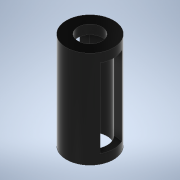
# Autodesk Inventor part: attachmentcustom
Saved by Autodesk Inventor 2022 (Build 260153000, 153)
## iProperties
Created: 2020-10-27
Part Number: attachmentcustom
Material: PET Plastic
Document SubType Name: Modeling
Designer: juanp
Density: 1.541 g/cm^3
Appearance: Polycarbonate - Clear
Author: juanp
Autodesk Inventor part; units mm, degrees
ref_plane "YZ Plane" through (0, 0, 0) normal (1, 0, 0) x (0, 1, 0)
ref_plane "XZ Plane" through (0, 0, 0) normal (0, 1, 0) x (-1, 0, 0)
ref_plane "XY Plane" through (0, 0, 0) normal (0, 0, 1) x (1, 0, 0)
sketch "Sketch6" plane through (0, 0, 0) normal (0, 1, 0) x (-1, 0, 0)
  circle A0 centre (0, 0) radius 8.75
  circle A1 centre (0, 0) radius 4.5
  dimension "d18" = 17.5
  dimension "d35" = 9
  constraints: 2 centre point, 2 coincident
  measures "d18" diameter of A0
  measures "d35" diameter of A1
extrude "Extrusion5" add sketch "Sketch6" along normal blind 36
sketch "Sketch10" plane through (0, 0, 0) normal (0, -1, 0) x (1, 0, 0)
  circle A0 centre (0, 0) radius 6.35
  dimension "d32" = 12.7
  constraints: 1 centre point, 1 coincident
  measures "d32" diameter of A0
extrude "Extrusion8" cut sketch "Sketch10" against normal blind 32.6
sketch "Sketch11" plane through (0, 32.6, 0) normal (0, -1, 0) x (1, 0, 0)
  arc A0 (-4.2968, -4.4) -> (4.2968, -4.4) centre (0, 0) ccw
  line L0 (-4.2968, 4.4) -> (-16.8146, 2.7257)
  arc A1 (-16.8146, 2.7257) -> (-16.8146, -2.7257) centre (-16.45, 0) ccw
  line L1 (-16.8146, -2.7257) -> (-4.2968, -4.4)
  line L2 (4.2968, -4.4) -> (16.8146, -2.7257)
  arc A2 (16.8146, -2.7257) -> (16.8146, 2.7257) centre (16.45, 0) ccw
  line L3 (16.8146, 2.7257) -> (4.2968, 4.4)
  line L4 (-4.2968, -4.4) -> (4.2968, -4.4) construction
  line L5 (-4.2968, 4.4) -> (4.2968, 4.4) construction
  line L6 (-19.2, 0) -> (19.2, 0) construction
  arc A3 (-6.15, 0) -> (-4.2968, -4.4) centre (0, 0) ccw construction
  arc A4 (-4.2968, 4.4) -> (-6.15, 0) centre (0, 0) ccw construction
  arc A5 (4.2968, 4.4) -> (-4.2968, 4.4) centre (0, 0) ccw
  arc A6 (6.15, 0) -> (4.2968, 4.4) centre (0, 0) ccw construction
  arc A7 (4.2968, -4.4) -> (6.15, 0) centre (0, 0) ccw construction
  line L7 (-4.3428, -4.4947) -> (-16.8278, -2.8248)
  arc A8 (-16.8278, 2.8248) -> (-16.8278, -2.8248) centre (-16.45, 0) ccw
  line L8 (-16.8278, 2.8248) -> (-4.3428, 4.4947)
  arc A9 (4.3428, 4.4947) -> (-4.3428, 4.4947) centre (0, 0) ccw
  line L9 (4.3428, 4.4947) -> (16.8278, 2.8248)
  arc A10 (16.8278, -2.8248) -> (16.8278, 2.8248) centre (16.45, 0) ccw
  line L10 (16.8278, -2.8248) -> (4.3428, -4.4947)
  arc A11 (-4.3428, -4.4947) -> (4.3428, -4.4947) centre (0, 0) ccw
  point P0 (0, 0)
  point P1 (0, 0)
  dimension "d36" = 12.3
  dimension "d37" = 8.8
  dimension "d38" = 38.4
  dimension "d39" = 2.75
  dimension "d40" = 0.1
  constraints: 30 point on circle, 22 end point, 12 centre point, 4 equal length, 4 tangent, 2 coincident, 2 horizontal, 2 point on line, 1 equal radius, 1 midpoint, 7 other
  measures "d36" diameter of A0
  measures "d37" distance between parallel lines of L5 L4
  measures "d38" distance of L6.start L6.end
  measures "d39" radius of A2
  measures "d40" distance between parallel lines of L1 L7
extrude "Extrusion9" cut sketch "Sketch11" along normal blind 29.2 contours L1 A1 L0 A5 L3 A2 L2 A0 | L7 A8 L8 A9 L9 A10 L10 A11
body "Solid2"
